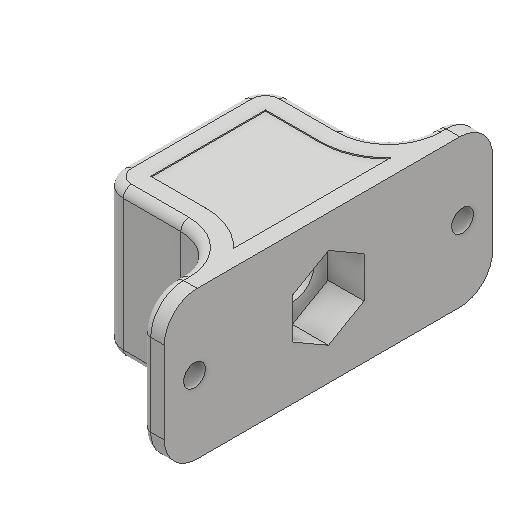
# Autodesk Inventor part: 3DP_ABS_Filament_Holder
Saved by Autodesk Inventor 2026.1 (Build 301233000, 233)
## iProperties
Created: 2016-06-28
Part Number: 3DP_ABS_Filament_Holder
Material: Ogólny
Document SubType Name: Modeling
Designer: Andrzej
Density: 1 g/cm^3
Appearance: Domyślna
Author: Andrzej
Autodesk Inventor part; units mm, degrees
ref_plane "YZ Plane" through (0, 0, 0) normal (1, 0, 0) x (0, 1, 0)
ref_plane "XZ Plane" through (0, 0, 0) normal (0, 1, 0) x (-1, 0, 0)
ref_plane "XY Plane" through (0, 0, 0) normal (0, 0, 1) x (1, 0, 0)
sketch "Szkic1" plane through (0, 0, 0) normal (0, 0, 1) x (1, 0, 0)
  line L0 (-23.1774, 10.5) -> (-23.1774, -19.5)
  line L1 (-23.1774, -19.5) -> (-0.6774, -19.5)
  line L2 (-0.6774, -19.5) -> (-0.6774, -34.5)
  line L3 (-0.6774, -34.5) -> (3.3226, -34.5)
  line L4 (3.3226, -34.5) -> (3.3226, 25.5)
  line L5 (3.3226, 25.5) -> (-0.6774, 25.5)
  line L6 (-23.1774, 10.5) -> (-0.6774, 10.5)
  line L7 (-0.6774, 25.5) -> (-0.6774, 10.5)
  point P0 (0, 0)
  dimension "d0" = 4
  dimension "d1" = 4
  dimension "d2" = 15
  dimension "d3" = 30
  dimension "d4" = 15
  dimension "d5" = 22.5
  constraints: 16 end point, 5 perpendicular, 2 vertical, 1 horizontal
  measures "d0" distance of L4.end L5.end
  measures "d1" distance of L2.end L3.end
  measures "d2" distance of L1.end L2.end
  measures "d3" distance of L0.start L0.end
  measures "d4" distance of L5.end L6.end
  measures "d5" distance of L0.start L6.end
extrude "Wyciągnięcie proste1" add sketch "Szkic1" along normal blind 27
sketch "Szkic2" plane through (3.3226, -34.5, 0) normal (1, 0, 0) x (0, 0, -1)
  line L0 (0, 0) -> (0, 60) projected
  line L1 (0, 60) -> (-27, 60) projected
  line L2 (-27, 0) -> (-27, 60) projected
  line L3 (0, 0) -> (-27, 0) projected
  circle A0 centre (-13.5, 30) radius 4
  line L4 (-9.7472, 36.5) -> (-5.9944, 30)
  line L5 (-5.9944, 30) -> (-9.7472, 23.5)
  line L6 (-9.7472, 23.5) -> (-17.2528, 23.5)
  line L7 (-17.2528, 23.5) -> (-21.0056, 30)
  line L8 (-21.0056, 30) -> (-17.2528, 36.5)
  line L9 (-17.2528, 36.5) -> (-9.7472, 36.5)
  point P0 (0, 34.5)
  point P1 (-13.5, 54.5)
  point P2 (-13.5, 5.5)
  point P3 (-13.5, 36.5)
  dimension "d8" = 27
  dimension "d9" = 13.5
  dimension "d11" = 13.5
  dimension "d12" = 5.5
  dimension "d13" = 5.5
  dimension "d14" = 60
  dimension "d16" = 8
  dimension "d18" = 30
  dimension "d43" = 6.5
  dimension "d44" = 7.5056
  dimension "d45" = 6.5
  dimension "d46" = 7.5056
  constraints: 12 end point, 1 centre point, 1 midpoint, 13 other
  measures "d8" distance of L0.end L1.end
  measures "d9" distance from line of L0 point (-13.5, 54.5)
  measures "d11" distance from line of L0 point (-13.5, 5.5)
  measures "d12" distance from line of L1 point (-13.5, 54.5)
  measures "d13" distance from line of L3 point (-13.5, 5.5)
  measures "d14" distance of L2.start L1.end
  measures "d16" diameter of A0
  measures "d18" distance from line of A0.centre L3
  measures "d43" distance of point (-13.5, 36.5) A0.centre
  measures "d44" distance of L7.end A0.centre
  measures "d45" distance from line of L6 A0.centre
  measures "d46" distance of L4.end A0.centre
hole "Otwór1" at (3.3226, 20, 13.5) at (3.3226, -29, 13.5) direction (-1, 0, 0) diameter 4 end through all
extrude "Wyciągnięcie proste2" cut sketch "Szkic2" against normal through all contours A0
sketch "Szkic3" plane through (-23.1774, -19.5, 0) normal (-1, 0, 0) x (0, 0, 1)
  circle A0 centre (13.5, 15) radius 4 projected
  line L0 (0, 30) -> (0, 0) projected
  line L1 (0, 0) -> (27, 0) projected
  line L2 (27, 30) -> (27, 0) projected
  line L3 (0, 30) -> (27, 30) projected
  circle A1 centre (13.5, 15) radius 10
  point P0 (0, 19.5)
  dimension "d28" = 20
  constraints: 1 centre point, 1 coincident
  measures "d28" diameter of A1
extrude "Wyciągnięcie proste3" cut sketch "Szkic3" against normal blind 6.4 contours A1
extrude "Wyciągnięcie proste4" cut sketch "Szkic2" against normal blind 6.6 contours L4 L5 L6 L7 L8 L9
fillet "Zaokrąglenie1" radius 6 4 edges at (1.3226, 25.5, 0) (1.3226, 25.5, 27) (1.3226, -34.5, 0) (1.3226, -34.5, 27)
fillet "Zaokrąglenie3" radius 8 2 edges at (-0.6774, 10.5, 13.5) (-0.6774, -19.5, 13.5)
fillet "Zaokrąglenie4" radius 4 2 edges at (-23.1774, 10.5, 13.5) (-23.1774, -19.5, 13.5)
sketch "Szkic4" plane through (-0.6774, -34.5, 6) normal (-1, 0, 0) x (0, 0, 1)
  circle A0 centre (7.5, 54.5) radius 2 projected
  circle A1 centre (7.5, 5.5) radius 2 projected
  circle A2 centre (7.5, 5.5) radius 2 projected
  circle A3 centre (7.5, 5.5) radius 5
  circle A4 centre (7.5, 54.5) radius 5
  point P0 (-6, 34.5)
  point P1 (6.1771, 53)
  point P2 (8.8229, 53)
  point P3 (8.8229, 7)
  point P4 (6.1771, 7)
  dimension "d38" = 10
  dimension "d39" = 10
  constraints: 2 centre point, 2 coincident
  measures "d38" diameter of A3
  measures "d39" diameter of A4
extrude "Wyciągnięcie proste5" cut sketch "Szkic4" along normal blind 4 contours A0 | A3 | A4
fillet "Zaokrąglenie5" radius 1.5 24 edges at (-22.0058, 9.3284, 0) (-23.1774, -4.5, 0) (-22.0058, -18.3284, 0) (-13.9274, -19.5, 0) (-3.0206, -21.8431, 0) (-0.6774, -28, 0) (-0.6774, -32.7426, 1.7574) (-0.6774, -34.5, 13.5) (-0.6774, -32.7426, 25.2426) (-0.6774, -28, 27) (-3.0206, -21.8431, 27) (-13.9274, -19.5, 27) (-22.0058, -18.3284, 27) (-23.1774, -4.5, 27) (-22.0058, 9.3284, 27) (-13.9274, 10.5, 27) (-3.0206, 12.8431, 27) (-0.6774, 19, 27) (-0.6774, 23.7426, 25.2426) (-0.6774, 25.5, 13.5) (-0.6774, 23.7426, 1.7574) (-0.6774, 19, 0) (-3.0206, 12.8431, 0) (-13.9274, 10.5, 0)
sketch "Szkic5" plane through (0, 0, 27) normal (0, 0, 1) x (1, 0, 0)
  line L0 (0.8226, -28.5) -> (0.8226, -27.5) projected
  line L1 (3.3226, -28.5) -> (0.8226, -28.5) projected
  line L2 (3.3226, -28.5) -> (3.3226, 19.5) projected
  line L3 (0.8226, 19.5) -> (3.3226, 19.5) projected
  line L4 (0.8226, 18.5) -> (0.8226, 19.5) projected
  arc A0 (-8.6774, 9) -> (0.8226, 18.5) centre (-8.6774, 18.5) ccw projected
  line L5 (-19.1774, 9) -> (-8.6774, 9) projected
  arc A1 (-19.1774, 9) -> (-21.6774, 6.5) centre (-19.1774, 6.5) ccw projected
  line L6 (-21.6774, -15.5) -> (-21.6774, 6.5) projected
  arc A2 (-21.6774, -15.5) -> (-19.1774, -18) centre (-19.1774, -15.5) ccw projected
  line L7 (-8.6774, -18) -> (-19.1774, -18) projected
  arc A3 (0.8226, -27.5) -> (-8.6774, -18) centre (-8.6774, -27.5) ccw projected
  line L8 (-8.6774, -15) -> (-18.6774, -15)
  line L9 (-18.6774, -15) -> (-18.6774, 6)
  line L10 (-18.6774, 6) -> (-8.6774, 6)
  arc A4 (-8.6774, 6) -> (0.3226, 9.8253) centre (-8.6774, 18.5) ccw
  line L11 (0.3226, 9.8253) -> (0.3226, -18.8253)
  arc A5 (0.3226, -18.8253) -> (-8.6774, -15) centre (-8.6774, -27.5) ccw
  point P0 (0, 0)
  dimension "d48" = 3
  constraints: 8 end point, 4 point on circle, 2 centre point, 2 other
  measures "d48" distance between parallel lines of L5 L10
extrude "Wyciągnięcie proste6" cut sketch "Szkic5" against normal blind 0.2 contours L8 L9 L10 A4 L11 A5
sketch "Szkic6" plane through (0, 0, 0) normal (0, 0, -1) x (-1, 0, 0)
  arc A0 (-0.3226, 9.8253) -> (8.6774, 6) centre (8.6774, 18.5) ccw projected
  line L0 (18.6774, 6) -> (8.6774, 6) projected
  line L1 (18.6774, -15) -> (18.6774, 6) projected
  line L2 (8.6774, -15) -> (18.6774, -15) projected
  arc A1 (8.6774, -15) -> (-0.3226, -18.8253) centre (8.6774, -27.5) ccw projected
  line L3 (-0.3226, 9.8253) -> (-0.3226, -18.8253) projected
  point P0 (0, 0)
extrude "Wyciągnięcie proste7" cut sketch "Szkic6" against normal blind 0.2
equation "\"d1\" = d0"
equation "\"d4\" = d2"
equation "\"d9\" = 0.5 * d8"
equation "\"d11\" = d9"
equation "\"d13\" = d12"
equation "\"d18\" = 0.5 * d14"
